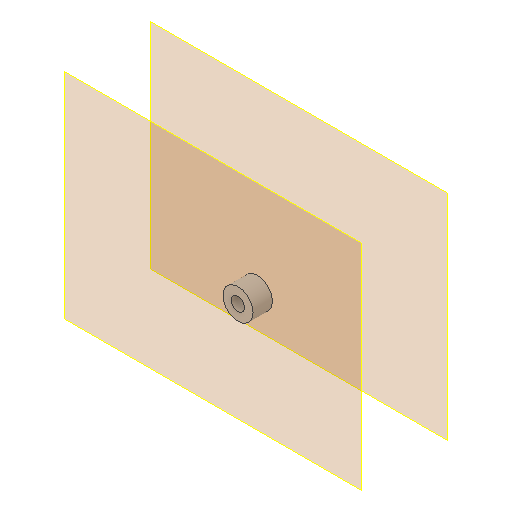
# Autodesk Inventor part: Neje_distancering
Saved by Autodesk Inventor 2022 (Build 260153000, 153)
## iProperties
Created: 2021-09-23
Part Number: Neje_distancering
Material: Generic
Document SubType Name: Modeling
Designer: diederichbenedict
Density: 1 g/cm^3
Appearance: Default
Author: diederichbenedict
Autodesk Inventor part; units mm, degrees
ref_plane "YZ Plane" through (0, 0, 0) normal (1, 0, 0) x (0, 1, 0)
ref_plane "XZ Plane" through (0, 0, 0) normal (0, 1, 0) x (-1, 0, 0)
ref_plane "XY Plane" through (0, 0, 0) normal (0, 0, 1) x (1, 0, 0)
ref_plane "Work Plane1" through (5.0077, 1.6686, 31) normal (0, 0, 1) x (-1, 0, 0)
ref_plane "Work Plane2" through (5.0077, 1.6686, 0) normal (0, 0, 1) x (1, 0, 0)
sketch "Sketch1" plane through (5.0077, 1.6686, 0) normal (0, 0, 1) x (1, 0, 0)
  circle A0 centre (-15.0077, -26.6686) radius 2.45 projected
  circle A1 centre (-15.0077, -26.6686) radius 5.45
  point P0 (-5.0077, -1.6686)
  dimension "d0" = 3
  constraints: 1 centre point
  measures "d0" radial gap between concentric circles of A0 A1
extrude "Extrusion1" add sketch "Sketch1" along normal blind 7
body "Solid1"
